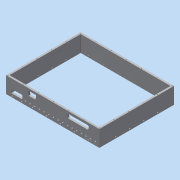
# Autodesk Inventor part: R58010-175-with SNAP V2 features
Saved by Autodesk Inventor 2016 (Build 200138000, 138)
## iProperties
Created: 2014-01-15
Part Number: R58010-175-with SNAP V2 features
Material: Aluminum 6061
Document SubType Name: Modeling
Designer: rtreacy
Density: 1 g/cm^3
Appearance: Aluminum - Flat
Vendor: Compac
Author: rtreacy
Autodesk Inventor part; units mm, degrees
note: some values were not read from the file. Chosen so that the rebuilt part matches the saved one: direction of "Hole_jackpost_dsub37"; direction of "Hole_jackpost_dsub9"; direction of "Hole26".
ref_plane "YZ Plane" through (0, 0, 0) normal (1, 0, 0) x (0, 1, 0)
ref_plane "XZ Plane" through (0, 0, 0) normal (0, 1, 0) x (-1, 0, 0)
ref_plane "XY Plane" through (0, 0, 0) normal (0, 0, 1) x (1, 0, 0)
sketch "Ext-Sketch" plane through (0, 0, 0) normal (0, 1, 0) x (-1, 0, 0)
  line L0 (-60.3663, -75.973) -> (184.1341, -75.973)
  line L1 (184.1341, -75.973) -> (184.1341, -269.6734)
  line L2 (184.1341, -269.6734) -> (-60.3663, -269.6734)
  line L3 (-60.3663, -269.6734) -> (-60.3663, -75.973)
  line L4 (188.8839, -274.4232) -> (-65.1161, -274.4232)
  line L5 (-65.1161, -274.4232) -> (-65.1161, -71.2232)
  line L6 (-65.1161, -71.2232) -> (188.8839, -71.2232)
  line L7 (188.8839, -71.2232) -> (188.8839, -274.4232)
  point P0 (0, 0)
  dimension "d6" = 244.5004
  dimension "d8" = 193.7004
  dimension "d9" = 203.2
  dimension "d10" = 254
  dimension "d11" = 4.7498
  dimension "d12" = 4.7498
  constraints: 16 end point, 4 parallel, 2 horizontal, 2 perpendicular
  measures "d6" distance of L0.start L0.end
  measures "d8" distance of L0.end L1.end
  measures "d9" distance of L6.end L4.start
  measures "d10" distance of L4.start L4.end
  measures "d11" horizontal distance of L0.start L5.end
  measures "d12" horizontal distance of L6.end L0.end
extrude "Extrusion1" add sketch "Ext-Sketch" along normal blind 44.45
sketch "left-2" plane through (-188.8839, 0, -274.4232) normal (-1, 0, 0) x (0, 0, 1)
  circle A0 centre (19.3548, 11.938) radius 2.1971 projected
  line L0 (203.2, 0) -> (0, 0) projected
  line L1 (203.2, 0) -> (203.2, 44.45) projected
  line L2 (0, 44.45) -> (203.2, 44.45) projected
  line L3 (0, 0) -> (0, 44.45) projected
  point P0 (274.4232, 0)
sketch "left-1" plane through (-188.8839, 0, -274.4232) normal (-1, 0, 0) x (0, 0, 1)
  line L0 (4.7498, 0) -> (4.7498, 44.45) projected
  point P0 (274.4232, 0)
  point P1 (203.2, 0)
  point P2 (203.2, 44.45)
  point P3 (158.75, 4.699)
  dimension "d260" = 44.45
  dimension "d261" = 4.699
  measures "d260" horizontal distance of point (203.2, 44.45) point (158.75, 4.699)
  measures "d261" vertical distance of point (203.2, 0) point (158.75, 4.699)
sketch "bottom-1" plane through (0, 0, 0) normal (0, -1, 0) x (1, 0, 0)
  point P0 (-188.8839, -71.2232)
  point P1 (0, 0)
  point P2 (-186.509, -73.5981)
  point P3 (65.1161, -274.4232)
  point P4 (62.7412, -272.0483)
  dimension "d125" = 2.3749
  dimension "d126" = 2.3749
  dimension "d140" = 2.3749
  dimension "d141" = 2.3749
  measures "d125" horizontal distance of point (-188.884, -71.223) point (-186.509, -73.598)
  measures "d126" horizontal distance of point (-188.884, -71.223) point (-186.509, -73.598)
  measures "d140" horizontal distance of point (65.116, -274.423) point (62.741, -272.048)
  measures "d141" horizontal distance of point (65.116, -274.423) point (62.741, -272.048)
hole "Hole8" at (-186.509, 0, -73.5981) direction (0, 1, 0) diameter 1.7018 depth 5.08 tip angle 118
hole "Hole9" at (62.7412, 0, -272.0483) direction (0, 1, 0) diameter 1.7018 depth 5.08 tip angle 118
sketch "front-1" plane through (-188.8839, 0, -71.2232) normal (0, 0, 1) x (1, 0, 0)
  circle A0 centre (52.07, 10.414) radius 2.159
  line L0 (254, 0) -> (254, 44.45) projected
  line L1 (14.2748, 19.746) -> (14.2748, 9.3472)
  line L2 (14.2748, 9.3472) -> (43.975, 9.3472)
  line L3 (43.975, 9.3472) -> (43.975, 19.746)
  line L4 (43.975, 19.746) -> (14.2748, 19.746)
  line L5 (0, 44.45) -> (254, 44.45) projected
  circle A1 centre (64.77, 10.414) radius 2.159
  circle A2 centre (77.47, 10.414) radius 2.159
  circle A3 centre (90.17, 10.414) radius 2.159
  circle A4 centre (102.87, 10.414) radius 2.159
  circle A5 centre (115.57, 10.414) radius 2.159
  circle A6 centre (128.27, 10.414) radius 2.159
  circle A7 centre (140.97, 10.414) radius 2.159
  circle A8 centre (153.67, 10.414) radius 2.159
  circle A9 centre (166.37, 10.414) radius 2.159
  circle A10 centre (179.07, 10.414) radius 2.159
  circle A11 centre (191.77, 10.414) radius 2.159
  circle A12 centre (204.47, 10.414) radius 2.159
  circle A13 centre (217.17, 10.414) radius 2.159
  circle A14 centre (229.87, 10.414) radius 2.159
  circle A15 centre (242.57, 10.414) radius 2.159
  point P0 (16.51, 4.699)
  point P1 (52.07, 16.51)
  point P2 (0, 0)
  point P3 (52.07, 4.318)
  point P4 (64.77, 16.51)
  point P5 (64.77, 4.318)
  point P6 (77.47, 16.51)
  point P7 (77.47, 4.318)
  point P8 (90.17, 16.51)
  point P9 (90.17, 4.318)
  point P10 (102.87, 16.51)
  point P11 (102.87, 4.318)
  point P12 (115.57, 16.51)
  point P13 (115.57, 4.318)
  point P14 (128.27, 16.51)
  point P15 (128.27, 4.318)
  point P16 (140.97, 16.51)
  point P17 (140.97, 4.318)
  point P18 (153.67, 16.51)
  point P19 (153.67, 4.318)
  point P20 (166.37, 16.51)
  point P21 (166.37, 4.318)
  point P22 (179.07, 16.51)
  point P23 (179.07, 4.318)
  point P24 (191.77, 16.51)
  point P25 (191.77, 4.318)
  point P26 (204.47, 16.51)
  point P27 (204.47, 4.318)
  point P28 (217.17, 16.51)
  point P29 (217.17, 4.318)
  point P30 (229.87, 16.51)
  point P31 (229.87, 4.318)
  point P32 (242.57, 16.51)
  point P33 (242.57, 4.318)
  point P34 (71.12, 4.699)
  dimension "d197" = 6.096
  dimension "d203" = 12.192
  dimension "d222" = 29.7002
  dimension "d223" = 10.3988
  dimension "d224" = 52.07
  dimension "d225" = 10.414
  dimension "d227" = 9.3472
  dimension "d259" = 4.699
  dimension "d273" = 12.7
  dimension "d299" = 14.2748
  dimension "d300" = 52.07
  dimension "d301" = 52.07
  dimension "d302" = 16.51
  dimension "d306" = 6.35
  dimension "d307" = 4.699
  dimension "d434" = 4.318
  constraints: 16 centre point, 8 end point, 3 parallel, 1 horizontal, 1 perpendicular, 60 other
  measures "d197" distance of point (52.07, 16.51) A0.centre
  measures "d203" distance of point (52.07, 16.51) point (52.07, 4.318)
  measures "d222" distance of L3.end L1.start
  measures "d223" distance of L2.end L3.end
  measures "d224" horizontal distance of L5.start A0.centre
  measures "d225" vertical distance of point (0, 0) A0.centre
  measures "d227" vertical distance of L0.start L2.end
  measures "d259" vertical distance of L0.start point (16.51, 4.699)
  measures "d273" distance of point (52.07, 16.51) point (64.77, 16.51)
  measures "d299" horizontal distance of L1.start L5.start
  measures "d300" horizontal distance of point (52.07, 16.51) L5.start
  measures "d301" horizontal distance of point (52.07, 4.318) L5.start
  measures "d302" horizontal distance of point (16.51, 4.699) point (0, 0)
  measures "d306" horizontal distance of point (71.12, 4.699) A1.centre
  measures "d307" vertical distance of point (0, 0) point (71.12, 4.699)
  measures "d434" diameter of A2
hole "Hole10" at (-172.3739, 4.699, -71.2232) direction (0, 0, -1) diameter 2.4384 depth 25.4 tip angle 118 countersink diameter 4.064 countersink angle 82
sketch "right-1" plane through (65.1161, 0, -71.2232) normal (1, 0, 0) x (0, 0, -1)
  point P0 (-71.2232, 0)
  point P1 (158.75, 4.699)
  point P2 (0, 0)
  point P3 (203.2, 44.45)
  dimension "d254" = 44.45
  dimension "d255" = 4.699
  measures "d254" horizontal distance of point (203.2, 44.45) point (158.75, 4.699)
  measures "d255" vertical distance of point (0, 0) point (158.75, 4.699)
hole "Hole11" at (65.1161, 4.699, -229.9732) direction (-1, 0, 0) diameter 2.4384 depth 25.4 tip angle 118 countersink diameter 4.064 countersink angle 82
sketch "back-1" plane through (65.1161, 0, -274.4232) normal (0, 0, -1) x (-1, 0, 0)
  point P0 (65.1161, 0)
  point P1 (228.6, 4.699)
  point P2 (254, 0)
  point P3 (254, 44.45)
  dimension "d256" = 25.4
  dimension "d257" = 4.699
  measures "d256" horizontal distance of point (254, 44.45) point (228.6, 4.699)
  measures "d257" vertical distance of point (254, 0) point (228.6, 4.699)
hole "Hole12" at (-163.4839, 4.699, -274.4232) direction (0, 0, 1) diameter 2.4384 depth 25.4 tip angle 118 countersink diameter 4.064 countersink angle 82
pattern_linear "Rectangular Pattern9" count 6 spacing 39.6748 along (0, 0, -1) of "Hole8"
pattern_linear "Rectangular Pattern10" count 7 spacing 41.529 along (1, 0, 0) of "Hole8"
pattern_linear "Rectangular Pattern11" count 6 spacing 39.6748 along (0, 0, 1) of "Hole9"
pattern_linear "Rectangular Pattern12" count 7 spacing 41.529 along (-1, 0, 0) of "Hole9"
sketch "top" plane through (0, 44.45, 0) normal (0, 1, 0) x (1, 0, 0)
  point P0 (-188.8839, 274.4232)
  point P1 (0, 0)
  point P2 (-186.4709, 272.0102)
  point P3 (65.1161, 184.1791)
  dimension "d176" = 2.413
  dimension "d177" = 2.413
  measures "d176" horizontal distance of point (-188.884, 274.423) point (-186.471, 272.01)
  measures "d177" horizontal distance of point (-188.884, 274.423) point (-186.471, 272.01)
hole "Hole13" at (-186.4709, 44.45, -272.0102) direction (0, -1, 0) diameter 1.7018 depth 5.08 tip angle 118
hole "Hole16" at (-136.8139, 16.51, -71.2232) at (-136.8139, 4.318, -71.2232) direction (0, 0, -1) diameter 1.7018 depth 25.4 tip angle 118
hole "Hole17" at (-136.8139, 10.414, -71.2232) direction (0, 0, -1) diameter 4.318 depth 25.4 tip angle 118
extrude "Extrusion2" cut sketch "front-1" against normal blind 25.4 contours L4 L3 L2 L1
hole "Hole18" at (-188.8839, 4.699, -115.6732) direction (1, 0, 0) diameter 2.4384 depth 25.4 tip angle 118 countersink diameter 4.064 countersink angle 82
hole "Hole19" at (-124.1139, 10.414, -71.2232) at (-111.4139, 10.414, -71.2232) at (-98.7139, 10.414, -71.2232) at (-86.0139, 10.414, -71.2232) at (-73.3139, 10.414, -71.2232) at (-60.6139, 10.414, -71.2232) at (-47.9139, 10.414, -71.2232) at (-35.2139, 10.414, -71.2232) at (-22.5139, 10.414, -71.2232) direction (0, 0, -1) diameter 4.318 depth 25.4 tip angle 118
hole "Hole20" at (-9.8139, 10.414, -71.2232) at (2.8861, 10.414, -71.2232) at (15.5861, 10.414, -71.2232) at (28.2861, 10.414, -71.2232) at (40.9861, 10.414, -71.2232) at (53.6861, 10.414, -71.2232) direction (0, 0, -1) diameter 4.318 depth 25.4 tip angle 118
hole "Hole21" at (-124.1139, 16.51, -71.2232) at (-124.1139, 4.318, -71.2232) at (-111.4139, 16.51, -71.2232) at (-111.4139, 4.318, -71.2232) at (-98.7139, 16.51, -71.2232) at (-98.7139, 4.318, -71.2232) at (-86.0139, 16.51, -71.2232) at (-86.0139, 4.318, -71.2232) at (-73.3139, 16.51, -71.2232) at (-73.3139, 4.318, -71.2232) at (-60.6139, 16.51, -71.2232) at (-60.6139, 4.318, -71.2232) at (-47.9139, 16.51, -71.2232) at (-47.9139, 4.318, -71.2232) at (-35.2139, 16.51, -71.2232) at (-35.2139, 4.318, -71.2232) at (-22.5139, 16.51, -71.2232) at (-22.5139, 4.318, -71.2232) at (-9.8139, 16.51, -71.2232) at (-9.8139, 4.318, -71.2232) at (2.8861, 16.51, -71.2232) at (2.8861, 4.318, -71.2232) at (15.5861, 16.51, -71.2232) at (15.5861, 4.318, -71.2232) at (28.2861, 16.51, -71.2232) at (28.2861, 4.318, -71.2232) at (40.9861, 16.51, -71.2232) at (40.9861, 4.318, -71.2232) at (53.6861, 16.51, -71.2232) at (53.6861, 4.318, -71.2232) direction (0, 0, -1) diameter 1.7018 depth 5.08 tip angle 118
pattern_linear "Rectangular Pattern13" count 2 spacing 25.4 along (1, 0, 0) of "Hole10"
hole "Hole22" at (-117.7639, 4.699, -71.2232) direction (0, 0, -1) diameter 2.4384 depth 25.4 tip angle 118 countersink diameter 4.064 countersink angle 82
pattern_linear "Rectangular Pattern14" count 5 spacing 38.1 along (1, 0, 0) of "Hole22"
pattern_linear "Rectangular Pattern15" count 6 spacing 40.64 along (1, 0, 0) of "Hole12"
pattern_linear "Rectangular Pattern16" count 4 spacing 38.1 along (0, 0, 1) of "Hole11"
pattern_linear "Rectangular Pattern17" count 4 spacing 38.1 along (0, 0, -1) of "Hole18"
pattern_linear "Rectangular Pattern19" count 6 spacing 39.6748 along (0, 0, 1) count 7 spacing 41.529 along (1, 0, 0) of "Hole13"
fillet "Fillet1" radius 1.524 1 edges at (-184.1341, 22.225, -269.6734)
fillet "Fillet2" radius 1.524 1 edges at (-184.1341, 22.225, -75.973)
fillet "Fillet3" radius 1.524 1 edges at (60.3663, 22.225, -75.973)
fillet "Fillet4" radius 1.524 1 edges at (60.3663, 22.225, -269.6734)
fillet "Fillet5" radius 0.7874 1 edges at (-174.6091, 9.3472, -73.5981)
fillet "Fillet6" radius 0.7874 1 edges at (-144.9089, 9.3472, -73.5981)
fillet "Fillet7" radius 0.7874 1 edges at (-144.9089, 19.746, -73.5981)
fillet "Fillet8" radius 0.7874 1 edges at (-174.6091, 19.746, -73.5981)
sketch "dsub37" plane through (-188.8839, 0, -71.2232) normal (0, 0, 1) x (1, 0, 0)
  line L0 (0, 44.45) -> (254, 44.45) projected
  circle A0 centre (227.6348, 32.512) radius 1.1303
  line L1 (254, 0) -> (254, 44.45) projected
  circle A1 centre (164.1348, 32.512) radius 1.1303
  line L2 (164.1348, 32.512) -> (227.6348, 32.512) construction
  line L3 (195.8848, 39.6875) -> (195.8848, 17.4625) construction
  line L4 (169.8244, 37.846) -> (221.9452, 37.846)
  line L5 (170.7007, 27.051) -> (221.0689, 27.051)
  line L6 (225.2236, 33.7907) -> (224.3473, 29.7013)
  line L7 (166.546, 33.7907) -> (167.4223, 29.7013)
  arc A2 (225.2236, 33.7907) -> (221.9452, 37.846) centre (221.9452, 34.4932) ccw
  arc A3 (221.0689, 27.051) -> (224.3473, 29.7013) centre (221.0689, 30.4038) ccw
  arc A4 (169.8244, 37.846) -> (166.546, 33.7907) centre (169.8244, 34.4932) ccw
  arc A5 (167.4223, 29.7013) -> (170.7007, 27.051) centre (170.7007, 30.4038) ccw
  line L8 (225.298, 34.4932) -> (225.298, 21.7627) construction
  point P0 (188.8839, 0)
  point P1 (195.8848, 32.512)
  point P2 (195.8848, 27.051)
  point P3 (195.8848, 37.846)
  dimension "d496" = 2.2606
  dimension "d497" = 26.3652
  dimension "d498" = 2.2606
  dimension "d499" = 63.5
  dimension "d504" = 50.3682
  dimension "d505" = 52.1208
  dimension "d506" = 3.3528
  dimension "d507" = 3.3528
  dimension "d508" = 3.3528
  dimension "d509" = 3.3528
  dimension "d510" = 5.334
  dimension "d511" = 10.795
  dimension "d544" = 11.938
  constraints: 14 end point, 9 tangent, 8 point on circle, 6 centre point, 3 midpoint, 3 point on line, 2 horizontal, 2 vertical
  measures "d496" diameter of A0
  measures "d497" distance from line of L1 L2.end
  measures "d498" diameter of A1
  measures "d499" distance of L2.end L2.start
  measures "d504" distance of A3.centre A5.centre
  measures "d505" distance of L4.start L4.end
  measures "d506" radius of A3
  measures "d507" radius of A2
  measures "d508" radius of A4
  measures "d509" radius of A5
  measures "d510" distance from line of L4 L2.start
  measures "d511" distance between parallel lines of L4 L5
  measures "d544" distance from line of L2.start L0
sketch "dsub9" plane through (-188.8839, 0, -71.2232) normal (0, 0, 1) x (1, 0, 0)
  circle A0 centre (58.42, 32.512) radius 1.1303
  circle A1 centre (83.4136, 32.512) radius 1.1303
  circle A2 centre (223.52, 4.699) radius 2.032 projected
  circle A3 centre (185.42, 4.699) radius 2.032 projected
  circle A4 centre (147.32, 4.699) radius 2.032 projected
  circle A5 centre (109.22, 4.699) radius 2.032 projected
  circle A6 centre (71.12, 4.699) radius 2.032 projected
  circle A7 centre (41.91, 4.699) radius 2.032 projected
  circle A8 centre (242.57, 16.51) radius 0.8509 projected
  circle A9 centre (229.87, 16.51) radius 0.8509 projected
  circle A10 centre (217.17, 16.51) radius 0.8509 projected
  circle A11 centre (204.47, 16.51) radius 0.8509 projected
  circle A12 centre (191.77, 16.51) radius 0.8509 projected
  circle A13 centre (179.07, 16.51) radius 0.8509 projected
  circle A14 centre (166.37, 16.51) radius 0.8509 projected
  circle A15 centre (153.67, 16.51) radius 0.8509 projected
  circle A16 centre (140.97, 16.51) radius 0.8509 projected
  circle A17 centre (128.27, 16.51) radius 0.8509 projected
  circle A18 centre (115.57, 16.51) radius 0.8509 projected
  circle A19 centre (102.87, 16.51) radius 0.8509 projected
  circle A20 centre (90.17, 16.51) radius 0.8509 projected
  circle A21 centre (77.47, 16.51) radius 0.8509 projected
  circle A22 centre (64.77, 16.51) radius 0.8509 projected
  circle A23 centre (64.77, 4.318) radius 0.8509 projected
  circle A24 centre (77.47, 4.318) radius 0.8509 projected
  circle A25 centre (90.17, 4.318) radius 0.8509 projected
  circle A26 centre (102.87, 4.318) radius 0.8509 projected
  circle A27 centre (115.57, 4.318) radius 0.8509 projected
  circle A28 centre (128.27, 4.318) radius 0.8509 projected
  circle A29 centre (140.97, 4.318) radius 0.8509 projected
  circle A30 centre (153.67, 4.318) radius 0.8509 projected
  circle A31 centre (166.37, 4.318) radius 0.8509 projected
  circle A32 centre (179.07, 4.318) radius 0.8509 projected
  circle A33 centre (191.77, 4.318) radius 0.8509 projected
  circle A34 centre (204.47, 4.318) radius 0.8509 projected
  circle A35 centre (217.17, 4.318) radius 0.8509 projected
  circle A36 centre (229.87, 4.318) radius 0.8509 projected
  circle A37 centre (242.57, 4.318) radius 0.8509 projected
  circle A38 centre (229.87, 10.414) radius 2.159 projected
  circle A39 centre (204.47, 10.414) radius 2.159 projected
  circle A40 centre (179.07, 10.414) radius 2.159 projected
  circle A41 centre (191.77, 10.414) radius 2.159 projected
  circle A42 centre (217.17, 10.414) radius 2.159 projected
  circle A43 centre (242.57, 10.414) radius 2.159 projected
  circle A44 centre (153.67, 10.414) radius 2.159 projected
  circle A45 centre (128.27, 10.414) radius 2.159 projected
  circle A46 centre (102.87, 10.414) radius 2.159 projected
  circle A47 centre (77.47, 10.414) radius 2.159 projected
  circle A48 centre (64.77, 10.414) radius 2.159 projected
  circle A49 centre (90.17, 10.414) radius 2.159 projected
  circle A50 centre (115.57, 10.414) radius 2.159 projected
  circle A51 centre (140.97, 10.414) radius 2.159 projected
  circle A52 centre (166.37, 10.414) radius 2.159 projected
  line L0 (43.1876, 9.3472) -> (15.0622, 9.3472) projected
  arc A53 (14.2748, 10.1346) -> (15.0622, 9.3472) centre (15.0622, 10.1346) ccw projected
  line L1 (14.2748, 10.1346) -> (14.2748, 18.9586) projected
  arc A54 (15.0622, 19.746) -> (14.2748, 18.9586) centre (15.0622, 18.9586) ccw projected
  line L2 (15.0622, 19.746) -> (43.1876, 19.746) projected
  arc A55 (43.975, 18.9586) -> (43.1876, 19.746) centre (43.1876, 18.9586) ccw projected
  line L3 (43.975, 18.9586) -> (43.975, 10.1346) projected
  arc A56 (43.1876, 9.3472) -> (43.975, 10.1346) centre (43.1876, 10.1346) ccw projected
  circle A57 centre (52.07, 10.414) radius 2.159 projected
  circle A58 centre (52.07, 16.51) radius 0.8509 projected
  circle A59 centre (52.07, 4.318) radius 0.8509 projected
  circle A60 centre (16.51, 4.699) radius 2.032 projected
  line L4 (254, 0) -> (0, 0) projected
  line L5 (254, 0) -> (254, 44.45) projected
  line L6 (0, 44.45) -> (254, 44.45) projected
  line L7 (0, 0) -> (0, 44.45) projected
  line L8 (58.42, 32.512) -> (83.4136, 32.512) construction
  line L9 (70.9168, 41.7782) -> (70.9168, 19.5407) construction
  line L10 (61.9252, 38.354) -> (79.9084, 38.354)
  line L11 (63.5127, 26.67) -> (78.3209, 26.67)
  arc A61 (78.3209, 26.67) -> (80.383, 28.3398) centre (78.3209, 28.7782) ccw
  arc A62 (81.9705, 35.8074) -> (79.9084, 38.354) centre (79.9084, 36.2458) ccw
  arc A63 (61.9252, 38.354) -> (59.8631, 35.8074) centre (61.9252, 36.2458) ccw
  arc A64 (61.4506, 28.3398) -> (63.5127, 26.67) centre (63.5127, 28.7782) ccw
  line L12 (59.8631, 35.8074) -> (61.4506, 28.3398)
  line L13 (81.9705, 35.8074) -> (80.383, 28.3398)
  line L14 (81.9705, 35.8074) -> (81.9705, 25.5688) construction
  line L15 (59.8631, 35.8074) -> (59.8631, 24.5456) construction
  point P0 (188.8839, 0)
  point P1 (70.9168, 32.512)
  point P2 (61.9768, 34.1382)
  point P3 (63.5127, 30.8864)
  point P4 (70.9168, 38.354)
  point P5 (70.9168, 26.67)
  dimension "d477" = 58.42
  dimension "d478" = 2.2606
  dimension "d479" = 2.2606
  dimension "d482" = 4.2164
  dimension "d483" = 4.2164
  dimension "d484" = 17.9832
  dimension "d485" = 14.8082
  dimension "d486" = 24.9936
  dimension "d490" = 5.842
  dimension "d491" = 11.684
  dimension "d492" = 4.2164
  dimension "d493" = 4.2164
  dimension "d545" = 11.938
  constraints: 16 end point, 10 point on circle, 8 tangent, 6 centre point, 3 horizontal, 3 midpoint, 3 point on line, 3 vertical
  measures "d477" distance from line of L8.start L7
  measures "d478" diameter of A0
  measures "d479" diameter of A1
  measures "d482" diameter of A63
  measures "d483" diameter of A64
  measures "d484" distance of A62.centre A63.centre
  measures "d485" distance of L11.start L11.end
  measures "d486" distance of L8.end L8.start
  measures "d490" distance from line of L10 L8.start
  measures "d491" distance between parallel lines of L11 L10
  measures "d492" diameter of A62
  measures "d493" diameter of A61
  measures "d545" distance from line of L8.start L6
hole "Hole_jackpost_dsub37" at (38.7509, 32.512, -71.2232) at (-24.7491, 32.512, -71.2232) direction (0, 0, -1) diameter 2.159 end up to surface
extrude "dsub37 cutout" cut sketch "dsub37" against normal up to surface (4.7498 mm away) contours L4 A2 L6 A3 L5 A5 L7 A4
hole "Hole_jackpost_dsub9" at (-105.4703, 32.512, -71.2232) at (-130.4639, 32.512, -71.2232) direction (0, 0, -1) diameter 2.159 end up to surface
extrude "dsub9 cutout" cut sketch "dsub9" against normal up to surface (4.7498 mm away) contours L10 A62 L13 A61 L11 A64 L12 A63
sketch "Sketch30" plane through (-188.8839, 0, -71.2232) normal (0, 0, 1) x (1, 0, 0)
  circle A0 centre (150.4442, 32.512) radius 1.9558 projected
  circle A1 centre (241.3254, 32.512) radius 1.9558 projected
  point P0 (188.8839, 0)
hole "Hole26" at (-38.4397, 32.512, -71.2232) at (52.4415, 32.512, -71.2232) direction (0, 0, -1) diameter 2.159 end up to surface
body "Solid1"
